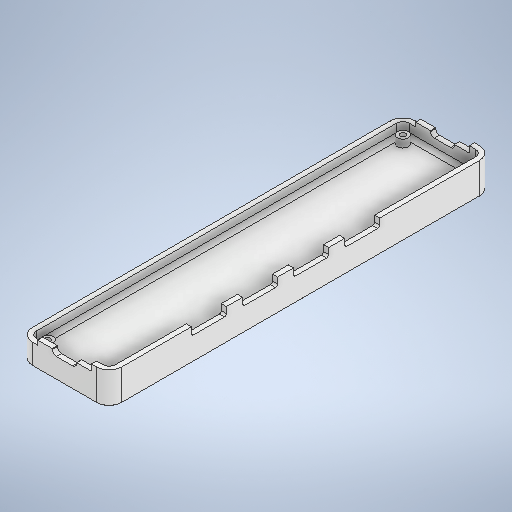
# Autodesk Inventor part: Lower_Housing
Saved by Autodesk Inventor 2025.1 (Build 291241020, 241B)
## iProperties
Created: 2026-01-18
Part Number: Lower_Housing
Material: Resina de poliariletercetona
Document SubType Name: Modeling
Designer: JoaoVitorRamosMitidi
Density: 1.32 g/cm^3
Appearance: Suave - Branco
Author: JoaoVitorRamosMitidi
Autodesk Inventor part; units mm, degrees
ref_plane "YZ Plane" through (0, 0, 0) normal (1, 0, 0) x (0, 1, 0)
ref_plane "XZ Plane" through (0, 0, 0) normal (0, 1, 0) x (-1, 0, 0)
ref_plane "XY Plane" through (0, 0, 0) normal (0, 0, 1) x (1, 0, 0)
sketch "Esboço1" plane through (0, 0, 0) normal (0, 1, 0) x (-1, 0, 0)
  line L0 (-13, 72.5) -> (13, 72.5)
  line L1 (15, 70.5) -> (15, -70.5)
  line L2 (13, -72.5) -> (-13, -72.5)
  line L3 (-15, -70.5) -> (-15, 70.5)
  line L4 (-15, 72.5) -> (15, -72.5) construction
  line L5 (15, 72.5) -> (-15, -72.5) construction
  circle A0 centre (12, 69.5) radius 1.1
  circle A1 centre (-12, 69.5) radius 1.1
  circle A2 centre (-12, -69.5) radius 1.1
  circle A3 centre (12, -69.5) radius 1.1
  circle A4 centre (-12, 69.5) radius 2.15
  circle A5 centre (12, 69.5) radius 2.15
  circle A6 centre (12, -69.5) radius 2.15
  circle A7 centre (-12, -69.5) radius 2.15
  arc A8 (15, 70.5) -> (13, 72.5) centre (13, 70.5) ccw
  arc A9 (-13, 72.5) -> (-15, 70.5) centre (-13, 70.5) ccw
  arc A10 (13, -72.5) -> (15, -70.5) centre (13, -70.5) ccw
  arc A11 (-15, -70.5) -> (-13, -72.5) centre (-13, -70.5) ccw
  circle A12 centre (-12, 69.5) radius 3.9
  circle A13 centre (12, 69.5) radius 3.9
  circle A14 centre (12, -69.5) radius 3.9
  circle A15 centre (-12, -69.5) radius 3.9
  point P0 (0, 0)
  dimension "d0" = 145
  dimension "d1" = 30
  dimension "d2" = 3
  dimension "d3" = 3
  dimension "d4" = 2.2
  dimension "d6" = 3
  dimension "d7" = 3
  dimension "d8" = 4.3
  dimension "d9" = 2
  dimension "d70" = 7.8
  constraints: 16 centre point, 12 end point, 12 equal radius, 8 coincident, 8 point on circle, 8 point on line, 8 tangent, 2 horizontal alignment, 2 midpoint, 2 parallel, 2 vertical alignment, 1 horizontal, 1 perpendicular
  measures "d0" distance of L5.start L4.end
  measures "d1" distance of L4.start L5.start
  measures "d2" distance from line of A1.centre L3
  measures "d3" distance from line of A1.centre L0
  measures "d4" diameter of A1
  measures "d6" distance from line of L1 A3.centre
  measures "d7" distance from line of L2 A3.centre
  measures "d8" diameter of A5
  measures "d9" radius of A8
  measures "d70" diameter of A12
extrude "Extrusão1" add sketch "Esboço1" along normal blind 3 contours L0 A12 L3 A9 | L0 A13 L1 A14 L2 A15 L3 A12 | L0 A8 L1 A13 | A15 L2 A11 L3 | L1 A10 L2 A14 | A0 | A1 | A2 | A3 | A4 | A5 | A6 | A7 picked at (-14.6958, 68.8312) picked at (14.6958, 68.8312) picked at (-14.6958, -68.8312) picked at (14.6958, -68.8312)
extrude "Extrusão3" add sketch "Esboço1" along normal blind 6 contours A4 | A5 | A6 | A7
extrude "Extrusão4" cut sketch "Esboço1" along normal blind 2 contours A4 | A5 | A6 | A7
extrude "Extrusão5" cut sketch "Esboço1" along normal up to surface (6 mm away) contours A0 | A1 | A2 | A3
sketch "Esboço3" plane through (0, 0, 0) normal (0, -1, 0) x (1, 0, 0)
  line L0 (13, -72.5) -> (-13, -72.5)
  line L1 (-15, -70.5) -> (-15, 70.5)
  line L2 (-13, 72.5) -> (13, 72.5)
  line L3 (15, 70.5) -> (15, -70.5)
  line L4 (15, -72.5) -> (-15, 72.5) construction
  line L5 (-15, -72.5) -> (15, 72.5) construction
  arc A0 (-15, -70.5) -> (-13, -72.5) centre (-13, -70.5) ccw
  arc A1 (13, -72.5) -> (15, -70.5) centre (13, -70.5) ccw
  arc A2 (15, 70.5) -> (13, 72.5) centre (13, 70.5) ccw
  arc A3 (-13, 72.5) -> (-15, 70.5) centre (-13, 70.5) ccw
  line L6 (12.5, -75) -> (-12.5, -75)
  line L7 (-17.5, -70) -> (-17.5, 70)
  line L8 (-12.5, 75) -> (12.5, 75)
  line L9 (17.5, 70) -> (17.5, -70)
  line L10 (17.5, -75) -> (-17.5, 75) construction
  line L11 (-17.5, -75) -> (17.5, 75) construction
  line L12 (13, -73) -> (-13, -73)
  line L13 (-15.5, -70.5) -> (-15.5, 70.5)
  line L14 (-13, 73) -> (13, 73)
  line L15 (15.5, 70.5) -> (15.5, -70.5)
  line L16 (15.5, -73) -> (-15.5, 73) construction
  line L17 (-15.5, -73) -> (15.5, 73) construction
  arc A4 (13, -73) -> (15.5, -70.5) centre (13, -70.5) ccw
  arc A5 (-15.5, -70.5) -> (-13, -73) centre (-13, -70.5) ccw
  arc A6 (-13, 73) -> (-15.5, 70.5) centre (-13, 70.5) ccw
  arc A7 (15.5, 70.5) -> (13, 73) centre (13, 70.5) ccw
  arc A8 (-17.5, -70) -> (-12.5, -75) centre (-12.5, -70) ccw
  arc A9 (12.5, -75) -> (17.5, -70) centre (12.5, -70) ccw
  arc A10 (17.5, 70) -> (12.5, 75) centre (12.5, 70) ccw
  arc A11 (-12.5, 75) -> (-17.5, 70) centre (-12.5, 70) ccw
  point P0 (0, 0)
  dimension "d20" = 145
  dimension "d21" = 30
  dimension "d22" = 2
  dimension "d23" = 2.5
  dimension "d24" = 2.5
  dimension "d25" = 31
  dimension "d26" = 146
  dimension "d27" = 2.5
  dimension "d30" = 5
  constraints: 36 end point, 24 point on circle, 24 point on line, 24 tangent, 12 centre point, 9 equal radius, 6 midpoint, 6 parallel, 3 horizontal, 3 perpendicular
  measures "d20" distance of L5.start L4.end
  measures "d21" distance between parallel lines of L1 L3
  measures "d22" radius of A0
  measures "d23" distance between parallel lines of L6 L0
  measures "d24" distance between parallel lines of L1 L7
  measures "d25" distance between parallel lines of L15 L13
  measures "d26" distance between parallel lines of L12 L14
  measures "d27" radius of A4
  measures "d30" radius of A8
extrude "Extrusão6" add sketch "Esboço3" against normal blind 3 contours L12 A5 L13 A6 L14 A7 L15 A4
extrude "Extrusão7" add sketch "Esboço3" against normal blind 7.682 contours L6 A8 L7 A11 L8 A10 L9 A9
sketch "Esboço4" plane through (0, 7.682, 0) normal (0, 1, 0) x (1, 0, 0)
  line L0 (-13, 73) -> (13, 73) projected
  line L1 (12.5, 75) -> (-12.5, 75) projected
  line L2 (-15.5, -70.5) -> (-15.5, 70.5) projected
  line L3 (-17.5, 70) -> (-17.5, -70) projected
  line L4 (13, -73) -> (-13, -73) projected
  line L5 (-12.5, -75) -> (12.5, -75) projected
  arc A0 (-17.5, -70) -> (-12.5, -75) centre (-12.5, -70) ccw projected
  arc A1 (-15.5, -70.5) -> (-13, -73) centre (-13, -70.5) ccw projected
  arc A2 (-12.5, 75) -> (-17.5, 70) centre (-12.5, 70) ccw projected
  arc A3 (-13, 73) -> (-15.5, 70.5) centre (-13, 70.5) ccw projected
  line L6 (-12.5, -75) -> (12.5, -75) projected
  arc A4 (12.5, -75) -> (17.5, -70) centre (12.5, -70) ccw projected
  line L7 (17.5, -70) -> (17.5, 70) projected
  arc A5 (17.5, 70) -> (12.5, 75) centre (12.5, 70) ccw projected
  line L8 (12.5, 75) -> (-12.5, 75) projected
  arc A6 (-12.5, 75) -> (-17.5, 70) centre (-12.5, 70) ccw projected
  line L9 (-17.5, 70) -> (-17.5, -70) projected
  arc A7 (-17.5, -70) -> (-12.5, -75) centre (-12.5, -70) ccw projected
  line L10 (15.5, 70.5) -> (15.5, -70.5) projected
  arc A8 (13, -73) -> (15.5, -70.5) centre (13, -70.5) ccw projected
  line L11 (13, -73) -> (-13, -73) projected
  arc A9 (-15.5, -70.5) -> (-13, -73) centre (-13, -70.5) ccw projected
  line L12 (-15.5, -70.5) -> (-15.5, 70.5) projected
  arc A10 (-13, 73) -> (-15.5, 70.5) centre (-13, 70.5) ccw projected
  line L13 (-13, 73) -> (13, 73) projected
  arc A11 (15.5, 70.5) -> (13, 73) centre (13, 70.5) ccw projected
  line L14 (10.5, 75) -> (10.5, 73)
  line L15 (10.5, -73) -> (10.5, -75)
  line L16 (-10.5, 73) -> (-10.5, 75)
  line L17 (-10.5, -75) -> (-10.5, -73)
  point P0 (0, 0)
  point P1 (10.5, -74)
  point P2 (12.5, 75)
  point P3 (12.5, -75)
  point P4 (-10.5, 74)
  dimension "d37" = 7
  dimension "d38" = 7
  dimension "d39" = 7
  constraints: 10 point on line, 8 end point, 3 perpendicular, 2 midpoint
  measures "d37" distance from line of L7 point (10.5, -74)
  measures "d38" distance from line of L3 point (-10.5, 74)
  measures "d39" distance between parallel lines of L3 L17
extrude "Extrusão8" add sketch "Esboço4" along normal blind 4.103 contours L14 L1 A5 L7 A4 L5 L15 L4 A8 L10 A11 L0
extrude "Extrusão9" add sketch "Esboço4" along normal blind 1.613 contours L16 L1 L14 L0
sketch "Esboço5" plane through (12.5, 0, -75) normal (0, 0, -1) x (-1, 0, 0)
  line L0 (2, 9.295) -> (23, 9.295) projected
  line L1 (7.83, 9.295) -> (7.83, 8.995)
  line L2 (9.31, 7.515) -> (15.69, 7.515)
  line L3 (17.17, 8.995) -> (17.17, 9.295)
  line L4 (23, 7.682) -> (23, 9.295) projected
  line L5 (25, 0) -> (0, 0) projected
  arc A0 (7.83, 8.995) -> (9.31, 7.515) centre (9.31, 8.995) ccw
  arc A1 (15.69, 7.515) -> (17.17, 8.995) centre (15.69, 8.995) ccw
  line L6 (2, 9.295) -> (2, 11.785) projected
  point P0 (12.5, 0)
  point P1 (3.25, 9.295)
  point P2 (17.17, 9.145)
  point P3 (3.25, 10.54)
  point P4 (7.83, 9.145)
  dimension "d42" = 9.34
  dimension "d44" = 5.83
  dimension "d45" = 7.515
  dimension "d46" = 1.48
  dimension "d57" = 5.83
  constraints: 6 end point, 4 point on circle, 4 tangent, 3 perpendicular, 2 centre point, 2 midpoint, 2 point on line, 1 equal radius, 1 other
  measures "d42" distance from line of point (17.17, 9.145) L1
  measures "d44" distance from line of L4 point (17.17, 9.145)
  measures "d45" distance between parallel lines of L5 L2
  measures "d46" radius of A0
extrude "Extrusão10" cut sketch "Esboço5" against normal up to surface (2 mm away)
extrude "Extrusão11" add sketch "Esboço4" along normal blind 1.688 contours L4 L15 L5 L17
sketch "Esboço6" plane through (-12.5, 0, 75) normal (0, 0, 1) x (1, 0, 0)
  line L0 (23, 9.37) -> (2, 9.37) projected
  line L1 (7.73, 9.37) -> (7.73, 9.07)
  line L2 (9.31, 7.49) -> (15.69, 7.49)
  line L3 (17.27, 9.07) -> (17.27, 9.37)
  line L4 (2, 7.682) -> (2, 9.37) projected
  arc A0 (7.73, 9.07) -> (9.31, 7.49) centre (9.31, 9.07) ccw
  arc A1 (15.69, 7.49) -> (17.27, 9.07) centre (15.69, 9.07) ccw
  point P0 (12.5, 0)
  point P1 (24.25, 9.37)
  point P2 (7.73, 7.49)
  point P3 (17.27, 7.49)
  point P4 (2, 8.526)
  dimension "d51" = 9.54
  dimension "d52" = 5.73
  dimension "d53" = 1.88
  dimension "d54" = 1.58
  constraints: 6 end point, 6 point on line, 4 point on circle, 4 tangent, 3 perpendicular, 2 centre point, 1 equal radius, 1 midpoint
  measures "d51" distance of point (7.73, 7.49) point (17.27, 7.49)
  measures "d52" distance from line of point (2, 8.526) L1
  measures "d53" distance between parallel lines of L0 L2
  measures "d54" radius of A0
extrude "Extrusão12" cut sketch "Esboço6" against normal up to surface (2 mm away)
sketch "Esboço7" plane through (17.5, 0, 70) normal (1, 0, 0) x (0, 0, -1)
  line L0 (140.5, 11.785) -> (-0.5, 11.785) projected
  line L1 (27.22, 11.785) -> (27.22, 9.425)
  line L2 (28.02, 8.625) -> (40.12, 8.625)
  line L3 (40.92, 9.425) -> (40.92, 11.785)
  line L4 (47.22, 11.785) -> (47.22, 9.425)
  line L5 (48.02, 8.625) -> (60.12, 8.625)
  line L6 (60.92, 9.425) -> (60.92, 11.785)
  line L7 (67.22, 11.785) -> (67.22, 9.425)
  line L8 (68.02, 8.625) -> (80.12, 8.625)
  line L9 (80.92, 9.425) -> (80.92, 11.785)
  line L10 (87.22, 11.785) -> (87.22, 9.425)
  line L11 (88.02, 8.625) -> (100.12, 8.625)
  line L12 (100.92, 9.425) -> (100.92, 11.785)
  line L13 (-5, 0) -> (-5, 11.785) projected
  line L14 (145, 0) -> (145, 11.785) projected
  arc A0 (27.22, 9.425) -> (28.02, 8.625) centre (28.02, 9.425) ccw
  arc A1 (40.12, 8.625) -> (40.92, 9.425) centre (40.12, 9.425) ccw
  arc A2 (47.22, 9.425) -> (48.02, 8.625) centre (48.02, 9.425) ccw
  arc A3 (60.12, 8.625) -> (60.92, 9.425) centre (60.12, 9.425) ccw
  arc A4 (67.22, 9.425) -> (68.02, 8.625) centre (68.02, 9.425) ccw
  arc A5 (80.12, 8.625) -> (80.92, 9.425) centre (80.12, 9.425) ccw
  arc A6 (87.22, 9.425) -> (88.02, 8.625) centre (88.02, 9.425) ccw
  arc A7 (100.12, 8.625) -> (100.92, 9.425) centre (100.12, 9.425) ccw
  point P0 (70, 0)
  point P1 (27.22, 8.625)
  point P2 (40.92, 8.625)
  point P3 (67.22, 8.625)
  point P4 (80.92, 8.625)
  point P5 (87.22, 8.625)
  point P6 (100.92, 8.625)
  dimension "d58" = 13.7
  dimension "d59" = 3.16
  dimension "d60" = 6.3
  dimension "d61" = 6.3
  dimension "d62" = 6.3
  dimension "d63" = 32.22
  dimension "d64" = 44.08
  dimension "d65" = 0.8
  constraints: 24 end point, 16 point on circle, 16 point on line, 16 tangent, 8 centre point, 7 equal radius, 6 vertical, 4 equal length, 3 perpendicular, 2 parallel, 9 other
  measures "d58" distance of point (27.22, 8.625) point (40.92, 8.625)
  measures "d59" distance of L1.start point (27.22, 8.625)
  measures "d60" distance between parallel lines of L4 L3
  measures "d61" distance between parallel lines of L7 L6
  measures "d62" distance between parallel lines of L10 L9
  measures "d63" distance between parallel lines of L13 L1
  measures "d64" distance between parallel lines of L14 L12
  measures "d65" radius of A0
extrude "Extrusão13" cut sketch "Esboço7" against normal up to surface (2 mm away)
fillet "Arredondamento1" radius 0.5 4 edges at (14.15, 0, 69.5) (-9.85, 0, 69.5) (-9.85, 0, -69.5) (14.15, 0, -69.5)
fillet "Arredondamento3" radius 1.5 8 edges at (-14.7678, 3, 72.2678) (0, 3, 73) (14.7678, 3, 72.2678) (15.5, 3, 0) (14.7678, 3, -72.2678) (0, 3, -73) (-14.7678, 3, -72.2678) (-15.5, 3, 0)
sketch "Esboço8" plane through (0, 0, 0) normal (0, -1, 0) x (1, 0, 0)
  circle A0 centre (-12, -69.5) radius 1.1 projected
  circle A1 centre (-12, -69.5) radius 2.65 projected
  line L0 (-12.5, -75) -> (12.5, -75) projected
  circle A2 centre (-12, -69.5) radius 2.65 projected
  circle A3 centre (12, 69.5) radius 2.65 projected
  line L1 (12.5, 75) -> (-12.5, 75) projected
  arc A4 (-12.5, 75) -> (-17.5, 70) centre (-12.5, 70) ccw projected
  line L2 (-17.5, 70) -> (-17.5, -70) projected
  arc A5 (-17.5, -70) -> (-12.5, -75) centre (-12.5, -70) ccw projected
  line L3 (-12.5, -75) -> (12.5, -75) projected
  arc A6 (12.5, -75) -> (17.5, -70) centre (12.5, -70) ccw projected
  line L4 (17.5, -70) -> (17.5, 70) projected
  arc A7 (17.5, 70) -> (12.5, 75) centre (12.5, 70) ccw projected
  circle A8 centre (-12, 69.5) radius 2.65 projected
  circle A9 centre (12, -69.5) radius 2.65 projected
  circle A10 centre (-12, -69.5) radius 4
  circle A11 centre (12, -69.5) radius 4
  circle A12 centre (12, 69.5) radius 4
  circle A13 centre (-12, 69.5) radius 4
  circle A14 centre (0, 0) radius 4
  dimension "d75" = 8
  dimension "d79" = 8
  constraints: 5 centre point, 5 coincident, 3 equal radius
  measures "d75" diameter of A13
  measures "d79" diameter of A14
extrude "Extrusão15" add sketch "Esboço8" along normal blind 0.5 contours A5 L2 A4 L1 A7 L4 A6 L0
fillet "Arredondamento5" radius 0.3 8 edges at (16.0355, -0.5, 73.5355) (0, -0.5, 75) (-16.0355, -0.5, 73.5355) (-17.5, -0.5, 0) (-16.0355, -0.5, -73.5355) (0, -0.5, -75) (16.0355, -0.5, -73.5355) (17.5, -0.5, 0)
